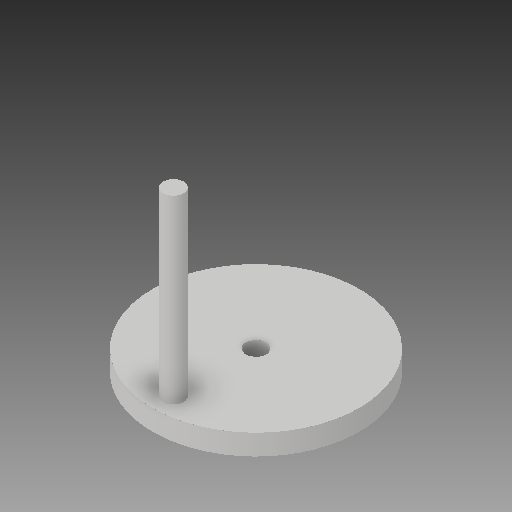
# Autodesk Inventor part: C1
Saved by Autodesk Inventor 2019 (Build 230136000, 136)
## iProperties
Created: 2020-03-27
Part Number: C1
Material: Generic
Document SubType Name: Modeling
Designer: Pulag
Density: 1 g/cm^3
Appearance: Default
Mass: 0.677013 g
Surface Area: 8.70221 cm^2
Volume: 0.677013 cm^3
Author: Pulag
Autodesk Inventor part; units mm, degrees
ref_plane "YZ Plane" through (0, 0, 0) normal (1, 0, 0) x (0, 1, 0)
ref_plane "XZ Plane" through (0, 0, 0) normal (0, 1, 0) x (-1, 0, 0)
ref_plane "XY Plane" through (0, 0, 0) normal (0, 0, 1) x (1, 0, 0)
sketch "Sketch1" plane through (0, 0, 0) normal (0, 1, 0) x (-1, 0, 0)
  circle A0 centre (0, 0) radius 10
  circle A1 centre (0, 8) radius 1
  dimension "d0" = 20
  dimension "d3" = 2
  constraints: 2 centre point, 1 coincident
  measures "d0" diameter of A0
  measures "d3" diameter of A1
sketch "Sketch2" plane through (0, 0, 0) normal (0, 1, 0) x (-1, 0, 0)
  circle A0 centre (0, 0) radius 10
  arc A1 (-5, 0) -> (5, 0) centre (0, 0) ccw
  arc A2 (-2.5, 0) -> (2.5, 0) centre (0, 0) ccw
  line L0 (5, 0) -> (2.5, 0)
  line L1 (-2.5, 0) -> (-5, 0)
  circle A3 centre (0, 8) radius 1
  circle A4 centre (0, 0) radius 1
  dimension "d4" = 20
  dimension "d5" = 10
  dimension "d6" = 5
  dimension "d7" = 2
  dimension "d12" = 2
  constraints: 5 centre point, 4 coincident, 4 end point, 4 point on circle, 2 horizontal
  measures "d4" diameter of A0
  measures "d5" diameter of A1
  measures "d6" diameter of A2
  measures "d7" diameter of A3
  measures "d12" diameter of A4
extrude "Extrusion2" add sketch "Sketch2" against normal blind 2 contours A0 | L1 A2 L0 A1 | A3
extrude "Extrusion3" add sketch "Sketch1" along normal blind 17.5 contours A1
body "Solid1"
